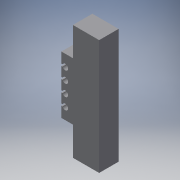
# Autodesk Inventor part: PiezaInferior
Saved by Autodesk Inventor 2017 (Build 210142000, 142)
## iProperties
Created: 2021-02-12
Part Number: PiezaInferior
Material: Generic
Document SubType Name: Modeling
Designer: USUARIO
Density: 1 g/cm^3
Appearance: Default
Author: USUARIO
Autodesk Inventor part; units mm, degrees
ref_plane "YZ Plane" through (0, 0, 0) normal (1, 0, 0) x (0, 1, 0)
ref_plane "XZ Plane" through (0, 0, 0) normal (0, 1, 0) x (-1, 0, 0)
ref_plane "XY Plane" through (0, 0, 0) normal (0, 0, 1) x (1, 0, 0)
sketch "Sketch3" plane through (0, 0, 0) normal (0, 1, 0) x (-1, 0, 0)
  line L0 (0, -300) -> (0, 0)
  line L1 (68.5, 0) -> (68.5, -75)
  line L2 (68.5, -75) -> (98.5, -75)
  line L3 (68.5, -300) -> (68.5, -225)
  line L4 (68.5, -225) -> (98.5, -225)
  line L5 (0, 0) -> (68.5, 0)
  line L6 (68.5, 0) -> (68.5, -75)
  line L7 (68.5, -75) -> (98.5, -75)
  line L8 (98.5, -75) -> (98.5, -225)
  line L9 (0, -300) -> (68.5, -300)
  circle A0 centre (88.5, -105) radius 7.5
  circle A1 centre (88.5, -135) radius 7.5
  circle A2 centre (88.5, -165) radius 7.5
  circle A3 centre (88.5, -195) radius 7.5
  dimension "d44" = 30
  dimension "d48" = 15
  dimension "d49" = 30
  dimension "d50" = 10
  dimension "d56" = 30
  dimension "d70" = 150
  dimension "d71" = 75
  dimension "d72" = 75
  dimension "d73" = 68.5
  dimension "d74" = 68.5
  dimension "d75" = 68.5
  dimension "d76" = 30
  dimension "d77" = 150
  dimension "d78" = 90
  dimension "d79" = 90
  constraints: 20 end point, 4 centre point, 2 collinear, 2 vertical, 1 horizontal, 6 other
  measures "d44" distance of L2.end L1.end
  measures "d48" diameter of A0
  measures "d49" distance from line of L2 A0.centre
  measures "d50" distance from line of A0.centre L8
  measures "d56" distance of A0.centre A1.centre
  measures "d70" distance of L2.end L4.end
  measures "d71" distance of L1.start L1.end
  measures "d72" distance of L3.start L3.end
  measures "d73" distance of L0.end L1.start
  measures "d74" distance of L0.start L3.start
  measures "d75" distance from line of L0 L3.end
  measures "d76" distance of L3.end L4.end
  measures "d77" distance of L1.end L3.end
  measures "d78" angle of L1 L2
  measures "d79" angle of L3 L4
extrude "Extrusion1" add sketch "Sketch3" along normal blind 50.8
sketch "Sketch6" plane through (0, 50.8, 0) normal (0, 1, 0) x (1, 0, 0)
  line L0 (-98.5, 225) -> (-98.5, 75) projected
  line L1 (-98.5, 102.5) -> (-95.5, 102.5)
  line L2 (-95.5, 102.5) -> (-95.5, 107.5)
  line L3 (-95.5, 107.5) -> (-98.5, 107.5)
  line L4 (-98.5, 107.5) -> (-98.5, 102.5)
  circle A0 centre (-88.5, 105) radius 7.5 projected
  line L5 (-95.5, 132.5) -> (-95.5, 137.5)
  line L6 (-95.5, 137.5) -> (-98.5, 137.5)
  line L7 (-98.5, 137.5) -> (-98.5, 132.5)
  line L8 (-98.5, 132.5) -> (-95.5, 132.5)
  line L9 (-95.5, 162.5) -> (-95.5, 167.5)
  line L10 (-95.5, 167.5) -> (-98.5, 167.5)
  line L11 (-98.5, 167.5) -> (-98.5, 162.5)
  line L12 (-98.5, 162.5) -> (-95.5, 162.5)
  line L13 (-95.5, 192.5) -> (-95.5, 197.5)
  line L14 (-95.5, 197.5) -> (-98.5, 197.5)
  line L15 (-98.5, 197.5) -> (-98.5, 192.5)
  line L16 (-98.5, 192.5) -> (-95.5, 192.5)
  point P0 (0, 0)
  dimension "d58" = 3
  dimension "d59" = 5
  dimension "d60" = 2.5
  dimension "d66" = 30
  constraints: 32 end point, 2 parallel, 1 horizontal, 1 perpendicular, 1 point on line, 1 vertical, 24 other
  measures "d58" distance of L3.end L2.end
  measures "d59" distance of L2.end L1.end
  measures "d60" distance from line of L1 A0.centre
  measures "d66" distance of L1.end L5.start
extrude "Extrusion3" cut sketch "Sketch6" against normal blind 50.8 contours L14 L13 L16 L0 | L10 L9 L12 L0 | L6 L5 L8 L0 | L3 A0 L1 L0 | L3 L2 L1 A0 picked at (-95.6506, 105.2826)
body "Solid1"
